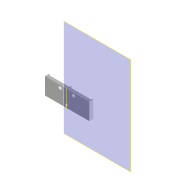
# Autodesk Inventor part: 00_cellSTORM_v5_chiptray_slidesize
Saved by Autodesk Inventor 2022 (Build 260153000, 153)
## iProperties
Created: 2020-05-10
Part Number: 00_cellSTORM_v5_chiptray_slidesize
Material: Generic
Document SubType Name: Modeling
Designer: diederichbenedict
Density: 1 g/cm^3
Appearance: Default
Author: diederichbenedict
Autodesk Inventor part; units mm, degrees
ref_plane "YZ Plane" through (0, 0, 0) normal (1, 0, 0) x (0, 1, 0)
ref_plane "XZ Plane" through (0, 0, 0) normal (0, 1, 0) x (-1, 0, 0)
ref_plane "XY Plane" through (0, 0, 0) normal (0, 0, 1) x (1, 0, 0)
ref_plane "Work Plane1" through (52.5141, 202.7033, 6.4479) normal (0, 0, -1) x (0, 1, 0)
sketch "Sketch1" plane through (52.5141, 202.7033, 6.4479) normal (0, 0, -1) x (0, 1, 0)
  circle A0 centre (-59.8114, -30.5) radius 2.95
  circle A1 centre (-38.8114, -18.3756) radius 2.95
  circle A2 centre (-38.8114, -42.6244) radius 2.95 construction
  circle A3 centre (-38.8114, -42.6244) radius 2.95
  line L0 (-38.8114, -42.6244) -> (-38.8114, -18.3756) construction
  line L1 (-38.8114, -18.3756) -> (-59.8114, -30.5) construction
  line L2 (-59.8114, -30.5) -> (-38.8114, -42.6244) construction
  line L3 (-63.9312, 9.5) -> (-63.9312, -70.5)
  line L4 (-63.9312, -70.5) -> (-33.9312, -70.5)
  line L5 (-33.9312, -70.5) -> (-33.9312, 9.5)
  line L6 (-33.9312, 9.5) -> (-63.9312, 9.5)
  line L7 (-63.9312, 9.5) -> (-33.9312, -70.5) construction
  line L8 (-63.9312, -70.5) -> (-33.9312, 9.5) construction
  point P0 (-202.7033, -52.5141)
  point P1 (-56.7146, -27.9576)
  point P2 (-59.6434, -27.5548)
  point P3 (-59.6434, -33.4452)
  dimension "d4" = 5.9
  dimension "d5" = 5.9
  dimension "d6" = 5.9
  dimension "d37" = 80
  dimension "d38" = 30
  constraints: 18 end point, 4 centre point, 2 parallel, 2 vertical, 1 coincident, 1 concentric, 1 perpendicular
  measures "d4" diameter of A0
  measures "d5" diameter of A1
  measures "d6" diameter of A2
  measures "d37" distance of L3.start L3.end
  measures "d38" distance of L4.end L3.end
extrude "Extrusion1" add sketch "Sketch1" along normal blind 4
sketch "Sketch2" plane through (52.5141, 202.7033, 2.4479) normal (0, 0, -1) x (-1, 0, 0)
  circle A0 centre (42.6244, -38.8114) radius 2.95 projected
  circle A1 centre (18.3756, -38.8114) radius 2.95 projected
  circle A2 centre (30.5, -59.8114) radius 2.95 projected
  line L0 (-9.5, -63.9312) -> (70.5, -63.9312) projected
  line L1 (70.5, -63.9312) -> (70.5, -33.9312) projected
  line L2 (70.5, -33.9312) -> (-9.5, -33.9312) projected
  line L3 (-9.5, -33.9312) -> (-9.5, -63.9312) projected
  point P0 (52.5141, -202.7033)
extrude "Extrusion2" add sketch "Sketch2" along normal blind 1.5 contours A0 | A1 | A2 | L3 L2 L1 L0
sketch "Skizze7" plane through (52.5141, 202.7033, 0.9479) normal (0, 0, -1) x (-1, 0, 0)
  line L0 (70.5, -63.9312) -> (70.5, -33.9312) projected
  line L1 (70.5, -33.9312) -> (-9.5, -33.9312) projected
  line L2 (-9.5, -33.9312) -> (-9.5, -63.9312) projected
  line L3 (-9.5, -63.9312) -> (70.5, -63.9312) projected
  line L4 (-8, -59.8091) -> (69, -59.8091)
  line L5 (69, -59.8091) -> (69, -33.8091)
  line L6 (69, -33.8091) -> (-8, -33.8091)
  line L7 (-8, -33.8091) -> (-8, -59.8091)
  line L8 (-8, -59.8091) -> (69, -33.8091) construction
  line L9 (69, -59.8091) -> (-8, -33.8091) construction
  line L10 (70.5, -33.9312) -> (-9.5, -33.9312) projected
  point P0 (52.5141, -202.7033)
  point P1 (30.5, -46.8091)
  point P2 (69, -33.9312)
  point P3 (-8, -33.9312)
  point P4 (69, -33.9312)
  dimension "d39" = 77
  dimension "d40" = 26
  constraints: 12 end point, 4 point on line, 2 midpoint, 2 parallel, 1 horizontal, 1 perpendicular
  measures "d39" distance of L6.end L5.end
  measures "d40" distance of L5.end L4.end
extrude "Extrusion7" add sketch "Skizze7" along normal blind 2 contours L3 L2 L1 L7 L4 L5 L0
ref_plane "Arbeitsebene2" through (22.0141, 138.7722, 6.4479) normal (-1, 0, 0) x (0, 0, 1)
body "Solid1"
